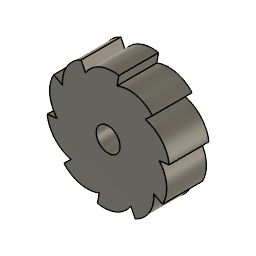
Ratchet (Autodesk Fusion 360 design; units mm, degrees)
part number: 2026-05-26-14-01-19-205
Autodesk Fusion 360 part; units mm, degrees
note: some values were not read from the file. Set by a fixed rule: which sketch regions a step uses.
sketch "ratchet" plane through (0, 0, 0) normal (0, 1, 0) x (1, 0, 0)
  circle A0 centre (0, 0) radius 6.5
  circle A1 centre (0, 0) radius 1.5
  circle A2 centre (0, 0) radius 2
  line L0 (0, 0) -> (1.3457, -7.6321)
  line L1 (0, 0) -> (-2.8494, -5.8422)
  arc A3 (-2.8494, -5.8422) -> (1.3457, -7.6321) centre (0.5378, -3.7146) ccw
  line L2 (0, 0) -> (7.7499, 0) construction
  arc A4 (1.3457, -7.6321) -> (0.8742, -7.7004) centre (0, 0) ccw
  dimension "d1" = 13
  dimension "d2" = 4
  dimension "d3" = 3
  dimension "d5" = 7.6321
  dimension "d6" = 36
  dimension "d7" = 4
  dimension "d12" = 80
  constraint coincident A0.centre A1.centre
  constraint coincident A0 L1.end
  constraint coincident L2.end A4
  constraint horizontal L2
  constraint concentric A0 A4
  constraint coincident A3 A4.end
  measures "d1" diameter of A0
  measures "d2" diameter of A2
  measures "d3" diameter of A1
  measures "d5" vertical distance of A0.centre L0.end
  measures "d6" angle of L0 L1
  measures "d7" radius of A3
  measures "d12" angle of L0 L2
extrude "Extrude1" add sketch "ratchet" against normal blind 5 contours A0 A2 L0 L1 | A0 L0 A3 picked at (-1.3488, -4.8046) makes body 1
pattern_circular "C-Pattern1" count 10 over 360 about axis through (0, -5, 0) along (0, 1, 0) of bodies 1 makes body 2 at (0.6078, -1.6667, 3.4468) makes body 3 at (7.548, -3.3333, 1.7247) makes body 4 at (7.1203, -3.3333, -3.0413) makes body 5 at (5.7473, -1.6667, -3.2337) makes body 6 at (-0.6922, -3.3333, -7.7116) makes body 7 at (-5.0927, -3.3333, -5.8319) makes body 8 at (-7.548, -3.3333, -1.7247) makes body 9 at (-7.1203, -3.3333, 3.0413) makes body 10 at (-1.5343, -1.6667, 3.1458)
extrude "Extrude2" add sketch "ratchet" against normal blind 5 contours A1 A2 L0 L1 | A1 A2 L0 L1 bodies 1 2 3 4 5 6 7 8 9 10
named bodies: "ratchet"
